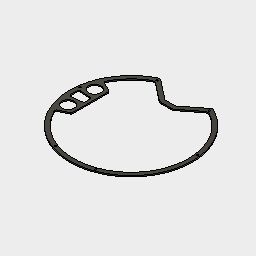
Top Plate (Autodesk Fusion 360 design; units mm, degrees)
Autodesk Fusion 360 part; units mm, degrees
sketch "Sketch1" plane through (0, 0, 0) normal (0, 1, 0) x (1, 0, 0)
  circle A0 centre (-85.0015, -22.7761) radius 10.5
  circle A1 centre (-85.0015, 22.7761) radius 10.5
  line L0 (-71.2336, 33.2168) -> (-86.0563, 40.1287)
  line L1 (-77.1365, 6.7486) -> (-94.5913, 8.2757)
  line L2 (-77.1374, -6.7486) -> (-94.5913, -8.2757)
  line L3 (-71.2336, -33.2168) -> (-86.0563, -40.1287)
  line L4 (-69.5015, 22.7761) -> (-69.5015, -22.7761)
  line L5 (-69.5015, 22.7761) -> (-69.5015, 30.4979)
  line L6 (-69.5015, -22.7761) -> (-69.5015, -30.4979)
  line L7 (-74.398, 3.7596) -> (-74.3988, -3.7604)
  arc A2 (-97.8481, 5.454) -> (-97.8481, -5.454) centre (0, 0) ccw
  arc A3 (-69.5015, 30.4979) -> (-71.2336, 33.2168) centre (-72.5015, 30.4979) ccw
  arc A4 (-87.466, 44.2007) -> (-86.0563, 40.1287) centre (-84.7884, 42.8476) ccw
  arc A5 (-94.5913, 8.2757) -> (-97.8481, 5.454) centre (-94.8528, 5.2871) ccw
  arc A6 (-97.8481, -5.454) -> (-94.5913, -8.2757) centre (-94.8528, -5.2871) ccw
  arc A7 (-77.1374, -6.7486) -> (-74.3988, -3.7604) centre (-77.3988, -3.7601) ccw
  arc A8 (-74.398, 3.7596) -> (-77.1365, 6.7486) centre (-77.398, 3.76) ccw
  arc A9 (-71.2336, -33.2168) -> (-69.5015, -30.4979) centre (-72.5015, -30.4979) ccw
  arc A10 (-86.0563, -40.1287) -> (-87.466, -44.2007) centre (-84.7884, -42.8476) ccw
  arc A11 (-46.4263, 94.1785) -> (46.4263, 94.1785) centre (0, 0) ccw
  arc A12 (-43.2519, 93.8511) -> (-46.4263, 94.1785) centre (-45.0998, 91.4877) ccw
  line L8 (-9.7255, 67.6367) -> (-43.2519, 93.8511)
  line L9 (7.8776, 67) -> (-7.8776, 67)
  line L10 (43.2519, 93.8511) -> (9.7255, 67.6367)
  arc A13 (46.4263, 94.1785) -> (43.2519, 93.8511) centre (45.0998, 91.4877) ccw
  arc A14 (-9.7255, 67.6367) -> (-7.8776, 67) centre (-7.8776, 70) ccw
  arc A15 (7.8776, 67) -> (9.7255, 67.6367) centre (7.8776, 70) ccw
  arc A16 (-46.4263, 94.1785) -> (46.4263, 94.1785) centre (0, 0) ccw
  arc A17 (-9.7255, 67.6367) -> (-7.8776, 67) centre (-7.8776, 70) ccw
  circle A18 centre (100.6317, 13.2484) radius 1.5
  circle A19 centre (-100.6317, 13.2484) radius 1.5
  circle A20 centre (-34.715, -95.3788) radius 1.5
  circle A21 centre (34.715, -95.3788) radius 1.5
  circle A22 centre (-44.8298, 89.3777) radius 1.55
  circle A23 centre (44.8298, 89.3777) radius 1.55
  line L11 (41.8995, 83.9078) -> (14.0372, 62.1222)
  arc A24 (7.8776, 60) -> (14.0372, 62.1222) centre (7.8776, 70) ccw
  line L12 (7.8776, 60) -> (-7.8776, 60)
  arc A25 (-14.0372, 62.1222) -> (-7.8776, 60) centre (-7.8776, 70) ccw
  line L13 (-14.0372, 62.1222) -> (-41.8995, 83.9078)
  arc A26 (-49.766, 84.4236) -> (-87.466, 44.2007) centre (0, 0) ccw
  arc A27 (-87.466, -44.2007) -> (49.766, 84.4236) centre (0, 0) ccw
  arc A28 (-41.8995, 83.9078) -> (-49.766, 84.4236) centre (-46.2112, 78.3934) ccw
  arc A29 (49.766, 84.4236) -> (41.8995, 83.9078) centre (46.2112, 78.3934) ccw
  dimension "d83" = 3
  dimension "d84" = 3
  dimension "d96" = 3
  dimension "d97" = 3
  measures "d83" diameter of A18
  measures "d84" diameter of A19
  measures "d96" diameter of A21
  measures "d97" diameter of A20
extrude "Extrude1" add sketch "Sketch1" along normal blind 2
